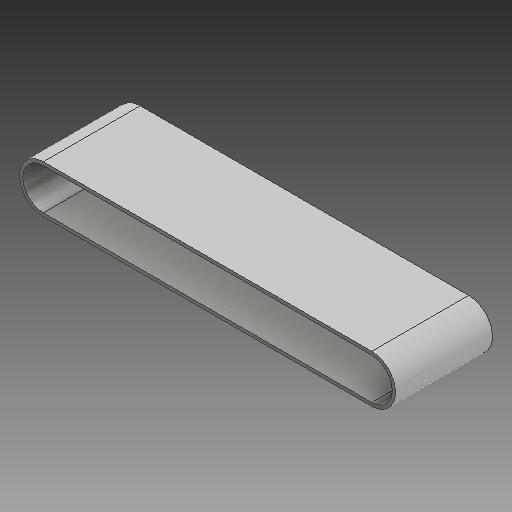
# Autodesk Inventor part: banda1
Saved by Autodesk Inventor 2019 (Build 230136000, 136)
## iProperties
Created: 2019-03-24
Part Number: banda1
Material: Generic
Document SubType Name: Modeling
Designer: felix
Density: 1 g/cm^3
Appearance: Default
Mass: 923.399 g
Surface Area: 3816.72 cm^2
Volume: 923.399 cm^3
Author: felix
Autodesk Inventor part; units mm, degrees
ref_plane "YZ Plane" through (0, 0, 0) normal (1, 0, 0) x (0, 1, 0)
ref_plane "XZ Plane" through (0, 0, 0) normal (0, 1, 0) x (-1, 0, 0)
ref_plane "XY Plane" through (0, 0, 0) normal (0, 0, 1) x (1, 0, 0)
sketch "Sketch1" plane through (0, 0, 0) normal (0, 0, 1) x (1, 0, 0)
  arc A0 (0, 31.75) -> (0, -31.75) centre (0, 0) ccw
  arc A1 (508, -31.75) -> (508, 31.75) centre (508, 0) ccw
  line L0 (508, -31.75) -> (25.9095, -31.75)
  line L1 (0, 31.75) -> (12.9547, 31.75)
  arc A2 (0, 36.75) -> (0, -36.75) centre (0, 0) ccw
  line L2 (0, 36.75) -> (508, 36.75)
  line L3 (508, -36.75) -> (0, -36.75)
  arc A3 (508, -36.75) -> (508, 36.75) centre (508, 0) ccw
  line L4 (495.0453, 31.75) -> (508, 31.75)
  line L5 (12.9547, 31.75) -> (495.0453, 31.75)
  line L6 (25.9095, -31.75) -> (0, -31.75)
  dimension "d0" = 63.5
  dimension "d1" = 508
  dimension "d2" = 73.5
  constraints: 14 end point, 11 tangent, 8 point on circle, 4 centre point, 2 concentric, 2 equal radius, 2 parallel, 1 coincident, 1 horizontal alignment
  measures "d0" diameter of A0
  measures "d1" distance of A1.centre A0.centre
  measures "d2" diameter of A2
extrude "Extrusion1" add sketch "Sketch1" along normal blind 150
body "Solid1"
